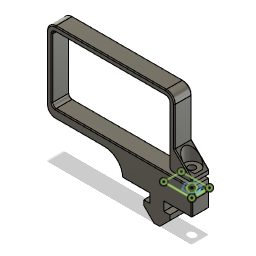
Shicks_PSU-clamp_Parametric (Autodesk Fusion 360 design; units mm, degrees)
Autodesk Fusion 360 part; units mm, degrees
sketch "Sketch1" plane through (0, 0, 0) normal (0, 0, 1) x (1, 0, 0)
  line L0 (20, 25.5) -> (0, 25.5) construction
  line L1 (0, 25.5) -> (0, 12) construction
  line L2 (14, 10.8) -> (14, 25.5)
  line L3 (6, 25.5) -> (14, 25.5)
  line L4 (6, 10.8) -> (6, 25.5) construction
  line L5 (8.3481, 2.2) -> (11.6519, 2.2)
  line L6 (6, 25.5) -> (6, 10.8)
  line L7 (30, 25.5) -> (-70, 25.5)
  line L8 (-48, 30.5) -> (30, 30.5)
  line L9 (30, 30.5) -> (30, 25.5)
  line L10 (20, 32.5) -> (19, 32.5)
  line L11 (17, 34.5) -> (17, 66.5)
  line L12 (20, 66.5) -> (20, 34.5)
  line L13 (-70, 25.5) -> (-53, 25.5)
  line L14 (-53, 25.5) -> (-53, 66.5)
  line L15 (-50, 66.5) -> (-50, 32.5)
  line L16 (-48, 68.5) -> (15, 68.5)
  line L17 (15, 71.5) -> (-48, 71.5)
  line L18 (20, 32.5) -> (30, 32.5)
  line L19 (30, 32.5) -> (30, 34.5)
  line L20 (30, 34.5) -> (20, 34.5)
  arc A0 (-48, 68.5) -> (-50, 66.5) centre (-48, 66.5) ccw
  arc A1 (17, 66.5) -> (15, 68.5) centre (15, 66.5) ccw
  arc A2 (-50, 32.5) -> (-48, 30.5) centre (-48, 32.5) ccw
  arc A3 (17, 34.5) -> (19, 32.5) centre (19, 34.5) ccw
  arc A4 (-48, 71.5) -> (-53, 66.5) centre (-48, 66.5) ccw
  arc A5 (20, 66.5) -> (15, 71.5) centre (15, 66.5) ccw
  line L21 (30, 25.5) -> (30, 15.5)
  line L22 (30, 15.5) -> (-10, 15.5)
  line L23 (-10, 15.5) -> (-10, 25.5)
  line L24 (2.5, 10.8) -> (2.5, 8.0481)
  line L25 (17.5, 10.8) -> (17.5, 8.0481)
  line L26 (2.5, 8.0481) -> (8.3481, 2.2)
  line L27 (17.5, 8.0481) -> (11.6519, 2.2)
  line L28 (17.5, 10.8) -> (14, 10.8)
  line L29 (2.5, 10.8) -> (6, 10.8)
  point P0 (0, 12)
  point P1 (17, 32.5)
  dimension "d2" = 13.5
  dimension "d3" = 8
  dimension "d5" = 6
  dimension "d10" = 14
  dimension "d12" = 5
  dimension "d13" = 3
  dimension "d16" = 30
  dimension "d22" = 10
  dimension "d23" = 2
  dimension "PSUWidth" = 67
  dimension "PSUHeight" = 38
  dimension "d30" = 3
  dimension "d31" = 3
  dimension "d32" = 2
  dimension "d36" = 30
  dimension "d40" = 2
  dimension "d56" = 3.3038
  dimension "d60" = 14.7
  dimension "d62" = 10
  dimension "d63" = 40
  constraint horizontal L0
  constraint vertical L1
  constraint coincident P0 L1.end
  constraint vertical L4
  constraint coincident L3.start L0
  constraint horizontal L7
  constraint vertical L9
  constraint coincident L0 L7.start
  constraint horizontal L10
  constraint horizontal L18
  constraint vertical L19
  constraint horizontal L20
  constraint tangent L15 A0
  constraint tangent L16 A0
  constraint tangent L16 A1
  constraint tangent L11 A1
  constraint tangent L8 A2
  constraint tangent L15 A2
  constraint coincident P1 L10
  constraint coincident P1 L11
  constraint tangent L10 A3
  constraint tangent L11 A3
  constraint concentric A0 A4
  constraint tangent L17 A4
  constraint concentric A1 A5
  constraint tangent L17 A5
  constraint perpendicular L7 L21
  constraint perpendicular L21 L22
  constraint coincident L7 L23.end
  constraint perpendicular L7 L23
  constraint perpendicular L0 L2
  constraint perpendicular L2 L28
  constraint perpendicular L6 L29
  constraint horizontal L24.start L25.start
  constraint horizontal L24.end L25.end
  constraint horizontal L5.end L5.start
  measures "d2" distance of L0.end P0
  measures "d3" distance of L3.start L2.end
  measures "d5" distance of L1 L4
  measures "d10" distance of origin L2
  measures "d12" distance of L7.start L8.end
  measures "d13" distance of L10.start P1
  measures "d16" distance of P0 L9
  measures "d22" distance of L10.start L18.end
  measures "d23" distance of L10.start L12.end
  measures "PSUWidth" distance of L11 L15
  measures "PSUHeight" distance of L8 L16
  measures "d30" distance of L14 L15
  measures "d31" distance of L16 L17
  measures "d32" radius of A0
  measures "d36" horizontal distance of P0 L18.end
  measures "d40" distance of L8 L18
  measures "d56" distance of L5.end L5.start
  measures "d60" distance of L4.start L3.start
  measures "d62" distance of L7.start L21.end
  measures "d63" distance of L21.end L22.end
extrude "Extrude1" add sketch "Sketch1" along normal blind 10
fillet "Fillet3" radius 5 1 edges at (-53, 25.5, 5)
chamfer "Chamfer1" distance 10 angle 45 1 edges at (20, 34.5, 5)
sketch "Sketch2" plane through (0, 30.5, 0) normal (0, 1, 0) x (-1, 0, 0)
  line L0 (-30, 0) -> (48, 0)
  line L1 (48, 0) -> (48, 10)
  line L2 (48, 10) -> (-30, 10)
  line L3 (-30, 10) -> (-30, 0)
  circle A0 centre (-25, 5) radius 4.5
  circle A1 centre (-25, 5) radius 2
  dimension "d38" = 9
  dimension "d39" = 4
  constraint concentric A0 A1
  measures "d38" diameter of A0
  measures "d39" diameter of A1
extrude "Extrude2" cut sketch "Sketch2" along normal blind 20 and the other way blind 20 contours A1
extrude "Extrude3" cut sketch "Sketch2" along normal blind 10 from surface at 5 contours A0
ref_plane "WorkPlane1" through (24.5, 25.5, 5) normal (0, -1, 0) x (1, 0, 0)
sketch "Sketch3" plane through (0, 25.5, 0) normal (0, -1, 0) x (1, 0, 0)
  line L0 (29.0414, 5.0056) -> (27.0159, 8.5028)
  line L1 (27.0159, 8.5028) -> (22.9744, 8.4972)
  line L2 (22.9744, 8.4972) -> (20.9586, 4.9944)
  line L3 (20.9586, 4.9944) -> (22.9841, 1.4972)
  line L4 (22.9841, 1.4972) -> (27.0256, 1.5028)
  line L5 (27.0256, 1.5028) -> (29.0414, 5.0056)
  circle A0 centre (25, 5) radius 2
  line L6 (14, 0) -> (30, 0)
  line L7 (30, 0) -> (30, 10)
  line L8 (30, 10) -> (14, 10)
  line L9 (14, 10) -> (14, 0)
  circle A1 centre (25, 5) radius 2
  line L10 (14, 0) -> (30, 0)
  line L11 (30, 0) -> (30, 10)
  line L12 (30, 10) -> (14, 10)
  line L13 (14, 10) -> (14, 0)
  circle A2 centre (25, 5) radius 2
  line L14 (14, 0) -> (30, 0)
  line L15 (30, 0) -> (30, 10)
  line L16 (30, 10) -> (14, 10)
  line L17 (14, 10) -> (14, 0)
  point P0 (25, 5)
  dimension "d48" = 3.5
  constraint coincident P0 A0.centre
  measures "d48" distance of P0 L5
extrude "Extrude4" cut sketch "Sketch3" along normal blind -2.5 and the other way blind 2 contours L0 L1 L2 L3 L4 L5
fillet "Fillet4" radius 10 1 edges at (-10, 25.5, 5)
chamfer "Chamfer2" distance 0.5 angle 45 40 edges at (-16.5, 71.5, 0) (18.5355, 70.0355, 0) (20, 55.5, 0) (-12.9289, 22.5711, 0) (-34, 25.5, 0) (-51.5355, 26.9645, 0) (-53, 48.5, 0) (-51.5355, 70.0355, 0) (25, 39.5, 0) (25, 39.5, 10) (30, 33.5, 10) (30, 33.5, 0) (30, 23, 0) (-34, 25.5, 10) (-51.5355, 26.9645, 10) (-53, 48.5, 10) (-51.5355, 70.0355, 10) (-16.5, 71.5, 10) (18.5355, 70.0355, 10) (20, 55.5, 10) (-12.9289, 22.5711, 10) (-9, 30.5, 10) (-49.4142, 31.0858, 10) (-50, 49.5, 10) (-49.4142, 67.9142, 10) (-16.5, 68.5, 10) (16.4142, 67.9142, 10) (17, 50.5, 10) (17.5858, 33.0858, 10) (24.5, 32.5, 10) (30, 23, 10) (-50, 49.5, 0) (-49.4142, 67.9142, 0) (-16.5, 68.5, 0) (16.4142, 67.9142, 0) (17, 50.5, 0) (17.5858, 33.0858, 0) (24.5, 32.5, 0) (-9, 30.5, 0) (-49.4142, 31.0858, 0)
chamfer "Chamfer2" distance 0.5 angle 45 6 edges at (30, 15.5, 5) (22, 15.5, 10) (22, 15.5, 0) (-2, 15.5, 0) (-10, 15.5, 5) (-2, 15.5, 10)
sketch "Sketch4" plane through (30, 0, 0) normal (1, 0, 0) x (0, 0, -1)
  line L0 (-9.5, 30.5) -> (-9.5, 16)
  line L1 (-0.5, 16) -> (-0.5, 30.5)
  line L2 (-0.5, 30.5) -> (-9.5, 30.5)
  line L3 (-1.5, 24) -> (-8.5, 24)
  line L4 (-8.5, 24) -> (-8.5, 28)
  line L5 (-8.5, 28) -> (-1.5, 28)
  line L6 (-1.5, 28) -> (-1.5, 24)
  line L7 (-1.5, 24) -> (-8.5, 28) construction
  line L8 (-8.5, 24) -> (-1.5, 28) construction
  line L9 (0, 25.5) -> (-10, 25.5)
  line L10 (-9.5, 16) -> (-0.5, 16)
  dimension "d68" = 7
  dimension "d69" = 4
  dimension "d70" = 2.5
  constraint horizontal L3
  constraint perpendicular L3 L4
  constraint parallel L3 L5
  constraint parallel L4 L6
  measures "d68" distance of L4.end L5.end
  measures "d69" distance of L3.end L4.end
  measures "d70" distance of L2 L5
extrude "Extrude5" cut sketch "Sketch4" against normal blind 5 contours L3 L4 L6 L9 | L4 L5 L6 L9
extrude "Extrude6" cut sketch "Sketch3" along normal blind 1.5 and the other way blind 2.5 contours L0 L1 L2 L3 L4 L5
equation "d1 = 20 mm"
equation "d5 = ( d1 - d3 ) / 2"
equation "d13 = d30"
equation "d31 = d30"
equation "d36 = d16"
equation "d60 = 4.70 mm + 10 mm"
